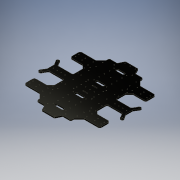
# Autodesk Inventor part: Acrylic Drivetrain Base - 1
Saved by Autodesk Inventor 2018 (Build 220112000, 112)
## iProperties
Created: 2018-08-24
Part Number: Acrylic Drivetrain Base - 1
Material: Generic
Document SubType Name: Modeling
Designer: anirudh
Density: 1 g/cm^3
Appearance: Gunmetal
Author: anirudh
Autodesk Inventor part; units mm, degrees
ref_plane "YZ Plane" through (0, 0, 0) normal (1, 0, 0) x (0, 1, 0)
ref_plane "XZ Plane" through (0, 0, 0) normal (0, 1, 0) x (-1, 0, 0)
ref_plane "XY Plane" through (0, 0, 0) normal (0, 0, 1) x (1, 0, 0)
sketch "Sketch1" plane through (0, 0, 0) normal (0, 1, 0) x (-1, 0, 0)
  line L0 (9.3096, -136.3312) -> (9.2955, -164.9037)
  circle A0 centre (71.6846, -205.4987) radius 1.85
  circle A1 centre (71.6846, -205.4987) radius 1.85
  circle A2 centre (156.9154, -205.4987) radius 1.85
  circle A3 centre (114.3, -205.4987) radius 1.85
  circle A4 centre (135.6077, -205.4987) radius 1.85
  circle A5 centre (92.9923, -205.4987) radius 1.85
  circle A6 centre (114.3, -256.2987) radius 1.85
  circle A7 centre (114.3, -307.0987) radius 1.85
  circle A8 centre (114.3, -357.8987) radius 1.85
  circle A9 centre (114.3, -403.3774) radius 1.85
  circle A10 centre (114.3, -205.4987) radius 1.85
  circle A11 centre (114.3, -154.6987) radius 1.85
  circle A12 centre (114.3, -103.8987) radius 1.85
  circle A13 centre (114.3, -53.0987) radius 1.85
  circle A14 centre (114.3, -7.62) radius 1.85
  circle A15 centre (31.75, -129.2987) radius 1.85
  circle A16 centre (31.75, -166.751) radius 1.85
  circle A17 centre (31.75, -92.7608) radius 1.85
  circle A18 centre (31.75, -281.6987) radius 1.85
  circle A19 centre (31.75, -244.2464) radius 1.85
  circle A20 centre (31.75, -318.2366) radius 1.85
  circle A21 centre (196.85, -129.2987) radius 1.85
  circle A22 centre (196.85, -166.751) radius 1.85
  circle A23 centre (196.85, -92.7608) radius 1.85
  circle A24 centre (196.85, -318.2366) radius 1.85
  circle A25 centre (196.85, -281.6987) radius 1.85
  circle A26 centre (196.85, -244.2464) radius 1.85
  line L1 (197.5093, -376.8271) -> (197.5095, -368.0768)
  line L2 (30.9869, -34.1675) -> (30.9883, -42.9178)
  line L3 (31.0103, -376.851) -> (31.011, -368.1007)
  line L4 (197.5254, -42.9116) -> (222.9296, -68.3074)
  line L5 (238.243, -117.2058) -> (219.1962, -136.2589)
  line L6 (219.1962, -274.5023) -> (238.2494, -293.5491)
  line L7 (222.9053, -342.6725) -> (197.5095, -368.0768)
  line L8 (5.6068, -342.705) -> (31.011, -368.1007)
  line L9 (-9.7544, -293.5747) -> (9.2924, -274.5216)
  line L10 (-9.7435, -117.2844) -> (9.3096, -136.3312)
  line L11 (5.5925, -68.322) -> (30.9883, -42.9178)
  arc A27 (158.3, -39.6917) -> (158.3, -43.3917) centre (158.3, -41.5417) ccw
  arc A28 (158.3, -167.6917) -> (158.3, -171.3917) centre (158.3, -169.5417) ccw
  circle A29 centre (139.7, -7.62) radius 1.85
  circle A30 centre (88.9, -7.62) radius 1.85
  circle A31 centre (139.7, -403.3774) radius 1.85
  circle A32 centre (88.9, -403.3774) radius 1.85
  circle A33 centre (156.9154, -182.6387) radius 1.85
  circle A34 centre (71.6846, -182.6387) radius 1.85
  circle A35 centre (156.9154, -228.3587) radius 1.85
  circle A36 centre (71.6846, -228.3587) radius 1.85
  circle A37 centre (144.8504, -332.4987) radius 1.85
  circle A38 centre (144.8504, -307.0987) radius 1.85
  circle A39 centre (144.8504, -281.6987) radius 1.85
  circle A40 centre (144.8504, -256.2987) radius 1.85
  circle A41 centre (144.8504, -354.6221) radius 1.85
  circle A42 centre (83.7496, -78.4987) radius 1.85
  circle A43 centre (83.7496, -103.8987) radius 1.85
  circle A44 centre (83.7496, -129.2987) radius 1.85
  circle A45 centre (83.7496, -154.6987) radius 1.85
  circle A46 centre (83.7496, -56.3753) radius 1.85
  circle A47 centre (83.7496, -281.6987) radius 1.85
  circle A48 centre (83.7496, -307.0987) radius 1.85
  circle A49 centre (83.7496, -332.4987) radius 1.85
  circle A50 centre (83.7496, -256.2987) radius 1.85
  circle A51 centre (196.85, -61.0108) radius 1.85
  circle A52 centre (196.85, -349.9866) radius 1.85
  circle A53 centre (31.75, -61.0108) radius 1.85
  circle A54 centre (31.75, -349.9866) radius 1.85
  arc A55 (124.9553, -184.4887) -> (124.9553, -180.7887) centre (124.9553, -182.6387) ccw
  arc A56 (124.9553, -230.2087) -> (124.9553, -226.5087) centre (124.9553, -228.3587) ccw
  arc A57 (103.6447, -180.7887) -> (103.6447, -184.4887) centre (103.6447, -182.6387) ccw
  arc A58 (103.6447, -226.5087) -> (103.6447, -230.2087) centre (103.6447, -228.3587) ccw
  line L12 (124.9553, -180.7887) -> (103.6447, -180.7887)
  line L13 (103.6447, -184.4887) -> (124.9553, -184.4887)
  line L14 (124.9553, -226.5087) -> (103.6447, -226.5087)
  line L15 (103.6447, -230.2087) -> (124.9553, -230.2087)
  circle A59 centre (222.9554, -81.0006) radius 1.85
  circle A60 centre (222.9554, -106.4006) radius 1.85
  circle A61 centre (205.7596, -112.7506) radius 1.85
  circle A62 centre (219.2568, -127.8041) radius 1.85
  circle A63 centre (222.9554, -329.9968) radius 1.85
  circle A64 centre (222.9554, -304.5968) radius 1.85
  circle A65 centre (205.7596, -298.2468) radius 1.85
  circle A66 centre (219.2568, -283.1933) radius 1.85
  circle A67 centre (5.6446, -81.0006) radius 1.85
  circle A68 centre (5.6446, -106.4006) radius 1.85
  circle A69 centre (22.8404, -112.7506) radius 1.85
  circle A70 centre (9.3432, -127.8041) radius 1.85
  circle A71 centre (22.8404, -298.2468) radius 1.85
  circle A72 centre (5.6446, -304.5968) radius 1.85
  circle A73 centre (5.6446, -329.9968) radius 1.85
  circle A74 centre (9.3432, -283.1933) radius 1.85
  circle A75 centre (15.5448, -164.846) radius 1.85
  circle A76 centre (15.5448, -246.1514) radius 1.85
  circle A77 centre (213.0552, -164.846) radius 1.85
  circle A78 centre (213.0552, -246.1514) radius 1.85
  line L16 (156.9471, -25.1432) -> (145.5867, -1.6614)
  arc A79 (197.5254, -34.1613) -> (191.1419, -27.8084) centre (191.1754, -34.1584) ccw
  arc A80 (145.5867, -1.6614) -> (142.9369, -0.0081) centre (142.9503, -2.9369) ccw
  arc A81 (156.9471, -25.1432) -> (160.8473, -27.8084) centre (161.2208, -23.0756) ccw
  line L17 (197.5093, -376.8271) -> (197.5095, -368.0768)
  line L18 (191.1555, -383.2007) -> (160.861, -383.2038)
  line L19 (156.961, -385.8694) -> (145.603, -409.3523)
  arc A82 (191.1555, -383.2007) -> (197.5093, -376.8271) centre (191.1593, -376.8507) ccw
  arc A83 (142.9534, -411.0059) -> (145.603, -409.3523) centre (142.9664, -408.0771) ccw
  arc A84 (160.861, -383.2038) -> (156.961, -385.8694) centre (161.2349, -387.9366) ccw
  line L20 (30.9869, -34.1675) -> (30.9883, -42.9178)
  line L21 (37.3358, -27.8164) -> (67.6304, -27.8114)
  line L22 (71.5302, -25.1455) -> (82.8866, -1.6618)
  arc A85 (37.3358, -27.8164) -> (30.9869, -34.1675) centre (37.3369, -34.1664) ccw
  arc A86 (85.5362, -0.0081) -> (82.8866, -1.6618) centre (85.5233, -2.9369) ccw
  arc A87 (67.6304, -27.8114) -> (71.5302, -25.1455) centre (67.2561, -23.0786) ccw
  arc A88 (31.0103, -376.851) -> (37.3598, -383.2016) centre (37.3603, -376.8516) ccw
  line L23 (37.3598, -383.2016) -> (67.6543, -383.2041)
  arc A89 (71.5543, -385.8697) -> (67.6543, -383.2041) centre (67.2805, -387.9369) ccw
  line L24 (71.5543, -385.8697) -> (82.9128, -409.3524)
  arc A90 (82.9128, -409.3524) -> (85.5625, -411.0059) centre (85.5493, -408.0771) ccw
  line L25 (9.2955, -164.9037) -> (9.2955, -171.2537)
  line L26 (5.5925, -68.322) -> (-60.4731, -68.322)
  line L27 (219.1962, -136.2589) -> (219.1962, -171.1839)
  line L28 (219.1962, -239.5772) -> (219.1962, -274.5023)
  line L29 (142.9534, -411.0059) -> (85.5625, -411.0059)
  line L30 (142.9369, -0.0081) -> (85.5362, -0.0081)
  line L31 (160.8473, -27.8084) -> (191.1419, -27.8084)
  line L32 (197.5254, -34.1613) -> (197.5254, -42.9116)
  line L33 (197.5254, -42.9116) -> (222.9296, -68.3074)
  line L34 (238.243, -117.2058) -> (219.2035, -136.2516)
  line L35 (-9.7435, -117.2844) -> (-61.6103, -117.2588)
  circle A91 centre (-85.9208, -164.4406) radius 1.85
  line L36 (-61.6103, -117.2588) -> (-37.1901, -117.2588) construction
  line L37 (-78.4107, -164.4544) -> (-65.7239, -184.4705)
  circle A92 centre (-85.9208, -246.5393) radius 1.85
  line L38 (-61.6326, -293.5491) -> (-37.2124, -293.5612) construction
  line L39 (-78.4057, -246.5412) -> (-65.7031, -226.5351)
  line L40 (-9.7544, -293.5747) -> (-61.6326, -293.5491)
  line L41 (-60.0894, -342.6725) -> (5.6068, -342.705)
  line L42 (-78.4057, -188.0789) -> (-78.4057, -222.901)
  line L43 (-91.143, -168.0218) -> (-78.4057, -188.0789)
  line L44 (-91.143, -242.9581) -> (-78.4057, -222.901)
  circle A93 centre (314.4543, -164.4406) radius 1.85
  line L45 (306.9417, -164.4412) -> (294.2391, -184.4473)
  line L46 (306.933, -246.5438) -> (294.2307, -226.5375)
  circle A94 centre (314.4543, -246.5393) radius 1.85
  line L47 (306.9392, -188.079) -> (306.9392, -222.901)
  line L48 (319.6764, -168.0218) -> (306.9392, -188.079)
  line L49 (319.6764, -242.9581) -> (306.9392, -222.901)
  line L50 (288.6229, -68.3074) -> (222.9296, -68.3074)
  line L51 (238.243, -117.2058) -> (290.1373, -117.2058)
  line L52 (290.1188, -293.5491) -> (238.2494, -293.5491)
  line L53 (222.9053, -342.6725) -> (288.6229, -342.6725)
  line L54 (-9.7435, -117.2844) -> (-61.6103, -117.2588)
  line L55 (-78.4107, -164.4544) -> (-65.7239, -184.4705)
  line L56 (-65.7031, -226.5351) -> (-78.4057, -246.5412)
  line L57 (-61.6326, -293.5491) -> (-9.7544, -293.5747)
  line L58 (238.243, -117.2058) -> (290.1373, -117.2058)
  line L59 (306.9417, -164.4412) -> (294.2391, -184.4473)
  line L60 (294.2307, -226.5375) -> (306.933, -246.5438)
  line L61 (290.1188, -293.5491) -> (238.2494, -293.5491)
  circle A95 centre (144.8375, -129.2857) radius 1.85
  circle A96 centre (144.8332, -103.8857) radius 1.85
  circle A97 centre (144.8289, -78.4857) radius 1.85
  circle A98 centre (144.8418, -154.6857) radius 1.85
  circle A99 centre (144.8251, -56.3623) radius 1.85
  arc A100 (159.225, -43.3917) -> (159.225, -39.6917) centre (159.225, -41.5417) ccw
  line L62 (159.225, -39.6917) -> (158.3, -39.6917)
  line L63 (158.3, -43.3917) -> (159.225, -43.3917)
  arc A101 (159.225, -171.3917) -> (159.225, -167.6917) centre (159.225, -169.5417) ccw
  line L64 (159.225, -167.6917) -> (158.3, -167.6917)
  line L65 (158.3, -171.3917) -> (159.225, -171.3917)
  arc A102 (158.3274, -367.5905) -> (158.328, -371.2905) centre (158.3277, -369.4405) ccw
  arc A103 (158.3058, -239.5905) -> (158.3064, -243.2905) centre (158.3061, -241.4405) ccw
  arc A104 (159.253, -371.2903) -> (159.2524, -367.5903) centre (159.2527, -369.4403) ccw
  line L66 (159.253, -371.2903) -> (158.328, -371.2905)
  line L67 (158.3274, -367.5905) -> (159.2524, -367.5903)
  arc A105 (159.2314, -243.2903) -> (159.2308, -239.5903) centre (159.2311, -241.4403) ccw
  line L68 (159.2314, -243.2903) -> (158.3064, -243.2905)
  line L69 (158.3058, -239.5905) -> (159.2308, -239.5903)
  arc A106 (70.2474, -43.3879) -> (70.2477, -39.6879) centre (70.2476, -41.5379) ccw
  arc A107 (70.2364, -171.3879) -> (70.2367, -167.6879) centre (70.2366, -169.5379) ccw
  arc A108 (69.3227, -39.6878) -> (69.3224, -43.3878) centre (69.3226, -41.5378) ccw
  line L70 (69.3227, -39.6878) -> (70.2477, -39.6879)
  line L71 (70.2474, -43.3879) -> (69.3224, -43.3878)
  arc A109 (69.3117, -167.6878) -> (69.3114, -171.3878) centre (69.3116, -169.5378) ccw
  line L72 (69.3117, -167.6878) -> (70.2367, -167.6879)
  line L73 (70.2364, -171.3879) -> (69.3114, -171.3878)
  line L74 (69.2988, -243.2864) -> (70.2238, -243.2867)
  arc A110 (69.2998, -239.5864) -> (69.2988, -243.2864) centre (69.2993, -241.4364) ccw
  line L75 (70.2248, -239.5867) -> (69.2998, -239.5864)
  arc A111 (69.2671, -367.5864) -> (69.2662, -371.2864) centre (69.2667, -369.4364) ccw
  line L76 (70.1921, -367.5867) -> (69.2671, -367.5864)
  line L77 (69.2662, -371.2864) -> (70.1912, -371.2867)
  arc A112 (70.2238, -243.2867) -> (70.2248, -239.5867) centre (70.2243, -241.4367) ccw
  arc A113 (70.1912, -371.2867) -> (70.1921, -367.5867) centre (70.1917, -369.4367) ccw
  line L78 (9.2955, -171.2537) -> (9.2955, -171.2643)
  line L79 (9.2924, -274.5216) -> (9.2924, -239.5943)
  circle A114 centre (-65.7031, -205.49) radius 1.85
  circle A115 centre (-46.6531, -205.49) radius 1.85
  circle A116 centre (-27.6031, -205.49) radius 1.85
  circle A117 centre (-8.5531, -205.49) radius 1.85
  circle A118 centre (294.2366, -205.5054) radius 1.85
  circle A119 centre (275.1866, -205.5038) radius 1.85
  circle A120 centre (256.1366, -205.5021) radius 1.85
  circle A121 centre (237.0866, -205.5005) radius 1.85
  line L80 (9.2924, -171.2627) -> (9.3096, -136.3312)
  line L81 (9.3096, -136.3312) -> (-9.7435, -117.2844)
  line L82 (-9.7435, -117.2844) -> (-61.6103, -117.2588)
  line L83 (-78.4107, -164.4544) -> (-65.7239, -184.4705)
  line L84 (9.2924, -171.2627) -> (9.3096, -136.3312)
  line L85 (-65.7696, -226.4913) -> (-78.4107, -246.5438)
  line L86 (-61.6326, -293.5491) -> (-9.7544, -293.5747)
  line L87 (-9.7544, -293.5747) -> (9.2924, -274.5216)
  line L88 (9.2924, -274.5216) -> (9.2924, -239.5943)
  line L89 (-60.4731, -68.322) -> (-61.6496, -68.322)
  line L90 (-71.1746, -77.847) -> (-71.1746, -107.7338)
  line L91 (-61.6496, -117.2588) -> (-61.6103, -117.2588)
  line L92 (-61.6496, -68.322) -> (-52.1246, -68.322)
  line L93 (-71.1746, -87.372) -> (-71.1746, -77.847)
  arc A122 (-61.6496, -68.322) -> (-71.1746, -77.847) centre (-61.6496, -77.847) ccw
  line L94 (-61.6496, -117.2588) -> (-52.1246, -117.2588)
  line L95 (-71.1746, -98.2088) -> (-71.1746, -107.7338)
  arc A123 (-71.1746, -107.7338) -> (-61.6496, -117.2588) centre (-61.6496, -107.7338) ccw
  line L96 (-87.0677, -156.6006) -> (-84.7607, -156.6006)
  line L97 (-78.4107, -162.9506) -> (-78.4107, -164.4544)
  line L98 (-87.0677, -254.3792) -> (-84.7607, -254.3792)
  line L99 (-78.4107, -248.0292) -> (-78.4107, -246.5438)
  line L100 (-71.1576, -303.0741) -> (-71.1576, -333.1475)
  line L101 (-60.0894, -342.6725) -> (-61.6326, -342.6725)
  line L102 (-61.6326, -293.5491) -> (-52.1076, -293.5491)
  line L103 (-71.1576, -312.5991) -> (-71.1576, -303.0741)
  line L104 (-61.6326, -342.6725) -> (-52.1076, -342.6725)
  line L105 (-71.1576, -323.6225) -> (-71.1576, -333.1475)
  arc A124 (-61.6279, -293.5491) -> (-71.1576, -303.0741) centre (-61.6326, -303.0741) ccw
  arc A125 (-71.1576, -333.1475) -> (-61.6326, -342.6725) centre (-61.6326, -333.1475) ccw
  line L106 (-65.7239, -184.4705) -> (2.9424, -184.4705)
  line L107 (9.2924, -178.1205) -> (9.2924, -171.2627)
  line L108 (-65.7696, -226.4913) -> (2.9424, -226.4913)
  line L109 (9.2924, -232.8413) -> (9.2924, -239.5943)
  line L110 (-93.0958, -164.9466) -> (-91.143, -168.0218)
  line L111 (-93.0958, -246.0333) -> (-91.143, -242.9581)
  line L112 (-87.0677, -156.6006) -> (-84.7607, -156.6006)
  line L113 (-87.0677, -156.6006) -> (-84.7607, -156.6006)
  arc A126 (-87.0677, -156.6006) -> (-93.0958, -164.9466) centre (-87.0677, -162.9506) ccw
  arc A127 (-78.4107, -162.9506) -> (-84.7607, -156.6006) centre (-84.7607, -162.9506) ccw
  line L114 (-78.4107, -246.5438) -> (-78.4107, -248.0292)
  arc A128 (-84.7607, -254.3792) -> (-78.4107, -248.0292) centre (-84.7607, -248.0292) ccw
  arc A129 (-93.0958, -246.0333) -> (-87.0677, -254.3792) centre (-87.0677, -248.0292) ccw
  line L115 (299.72, -326.2376) -> (299.72, -333.1475)
  line L116 (290.195, -342.6725) -> (288.6229, -342.6725)
  line L117 (299.72, -326.2376) -> (299.72, -303.0741)
  line L118 (290.195, -293.5491) -> (290.1188, -293.5491)
  line L119 (290.195, -342.6725) -> (280.67, -342.6725)
  line L120 (299.72, -323.6225) -> (299.72, -333.1475)
  arc A130 (290.195, -342.6725) -> (299.72, -333.1475) centre (290.195, -333.1475) ccw
  line L121 (290.195, -293.5491) -> (280.67, -293.5491)
  line L122 (299.72, -312.5991) -> (299.72, -303.0741)
  arc A131 (299.72, -303.0741) -> (290.195, -293.5491) centre (290.195, -303.0741) ccw
  line L123 (290.1373, -117.2058) -> (290.1994, -117.2058)
  line L124 (299.7244, -107.6808) -> (299.7244, -77.8324)
  line L125 (290.195, -68.3074) -> (288.6229, -68.3074)
  line L126 (290.1994, -117.2058) -> (280.6744, -117.2058)
  line L127 (299.7244, -98.1558) -> (299.7244, -107.6808)
  line L128 (290.195, -68.3074) -> (280.67, -68.3074)
  line L129 (299.7244, -87.3574) -> (299.7244, -77.8324)
  arc A132 (290.1994, -117.2058) -> (299.7244, -107.6808) centre (290.1994, -107.6808) ccw
  arc A133 (299.7244, -77.8324) -> (290.195, -68.3074) centre (290.1994, -77.8324) ccw
  line L130 (294.2307, -226.5375) -> (225.5462, -226.5375)
  line L131 (219.1962, -232.8875) -> (219.1962, -239.5772)
  line L132 (294.2391, -184.4473) -> (225.5462, -184.4473)
  line L133 (219.1962, -178.0973) -> (219.1962, -171.1839)
  line L134 (315.6011, -254.3793) -> (313.283, -254.3793)
  line L135 (306.933, -248.0293) -> (306.933, -246.5438)
  line L136 (321.6293, -246.0333) -> (319.6764, -242.9581)
  line L137 (306.9417, -164.4412) -> (306.9417, -162.968)
  line L138 (313.2917, -156.618) -> (315.6012, -156.618)
  line L139 (321.6411, -164.9279) -> (319.6764, -168.0218)
  arc A134 (315.6011, -254.3793) -> (321.6293, -246.0333) centre (315.6011, -248.0293) ccw
  line L140 (313.283, -254.3793) -> (315.6011, -254.3793)
  line L141 (306.933, -246.5438) -> (306.933, -248.0293)
  arc A135 (306.933, -248.0293) -> (313.283, -254.3793) centre (313.283, -248.0293) ccw
  line L142 (315.6012, -156.618) -> (313.2917, -156.618)
  arc A136 (321.6411, -164.9279) -> (315.6012, -156.618) centre (315.6012, -162.968) ccw
  line L143 (313.2917, -156.618) -> (315.6012, -156.618)
  line L144 (306.9417, -164.4412) -> (306.9417, -162.968)
  arc A137 (313.2917, -156.618) -> (306.9417, -162.968) centre (313.2917, -162.968) ccw
  line L145 (2.9424, -184.4705) -> (-3.4076, -184.4705)
  line L146 (9.2924, -171.7705) -> (9.2924, -178.1205)
  arc A138 (2.9424, -184.4705) -> (9.2924, -178.1205) centre (2.9424, -178.1205) ccw
  line L147 (2.9424, -226.4913) -> (-3.4076, -226.4913)
  line L148 (9.2924, -239.1913) -> (9.2924, -232.8413)
  arc A139 (9.2924, -232.8413) -> (2.9424, -226.4913) centre (2.9424, -232.8413) ccw
  line L149 (225.5462, -184.4473) -> (231.8962, -184.4473)
  line L150 (219.1962, -171.7473) -> (219.1962, -178.0973)
  line L151 (225.5462, -226.5375) -> (231.8962, -226.5375)
  line L152 (219.1962, -239.2375) -> (219.1962, -232.8875)
  arc A140 (219.1962, -178.0973) -> (225.5462, -184.4473) centre (225.5462, -178.0973) ccw
  arc A141 (225.5462, -226.5375) -> (219.1962, -232.8875) centre (225.5462, -232.8875) ccw
  circle A142 centre (196.85, -205.4987) radius 1.85
  circle A143 centre (31.75, -205.4987) radius 1.85
  circle A144 centre (290.195, -84.7598) radius 2.032
  circle A145 centre (290.195, -100.7618) radius 2.032
  circle A146 centre (258.191, -84.7598) radius 2.032
  circle A147 centre (258.191, -100.7618) radius 2.032
  circle A148 centre (290.195, -310.2356) radius 2.032
  circle A149 centre (290.195, -326.2376) radius 2.032
  circle A150 centre (258.191, -310.2356) radius 2.032
  circle A151 centre (258.191, -326.2376) radius 2.032
  circle A152 centre (-29.591, -310.2356) radius 2.032
  circle A153 centre (-29.591, -326.2376) radius 2.032
  circle A154 centre (-61.6085, -310.2203) radius 2.032
  circle A155 centre (-61.6106, -326.2223) radius 2.032
  circle A156 centre (-29.591, -84.7598) radius 2.032
  circle A157 centre (-29.591, -100.7618) radius 2.032
  circle A158 centre (-61.6106, -84.7576) radius 2.032
  circle A159 centre (-61.6085, -100.7596) radius 2.032
  circle A160 centre (83.7496, -354.6221) radius 1.85
  constraints: 306 end point, 161 centre point, 104 point on circle, 32 horizontal, 25 perpendicular, 17 collinear, 9 parallel, 8 vertical, 7 tangent, 2 point on line
ref_plane "Work Plane2" through (0, 6.35, 0) normal (0, 1, 0) x (1, 0, 0)
extrude "Extrusion21" add sketch "Sketch1" along normal blind 5.588
sketch "Sketch4" plane through (0, 5.588, 0) normal (0, 1, 0) x (1, 0, 0)
  circle A0 centre (-144.8251, 56.3623) radius 1.85 projected
  circle A1 centre (-83.7496, 56.3753) radius 1.85 projected
  circle A2 centre (-144.8418, 154.6857) radius 1.85 projected
  circle A3 centre (-83.7496, 154.6987) radius 1.85 projected
  circle A4 centre (-144.8504, 256.2987) radius 1.85 projected
  circle A5 centre (-83.7496, 256.2987) radius 1.85 projected
  circle A6 centre (-83.7496, 354.6221) radius 1.85 projected
  circle A7 centre (-144.8504, 354.6221) radius 1.85 projected
  arc A8 (-129.5313, 62.7155) -> (-129.5313, 50.0156) centre (-129.5532, 56.3656) ccw
  arc A9 (-99.0384, 50.0156) -> (-99.0384, 62.7155) centre (-99.0165, 56.3656) ccw
  arc A10 (-129.5313, 161.0421) -> (-129.5313, 148.3423) centre (-129.5709, 154.6922) ccw
  arc A11 (-99.0624, 148.3423) -> (-99.0624, 161.0421) centre (-99.0228, 154.6922) ccw
  arc A12 (-129.5313, 262.6485) -> (-129.5313, 249.9489) centre (-129.5752, 256.2987) ccw
  arc A13 (-99.0687, 249.9489) -> (-99.0687, 262.6485) centre (-99.0248, 256.2987) ccw
  arc A14 (-129.5313, 360.9719) -> (-129.5752, 348.2721) centre (-129.5752, 354.6221) ccw
  arc A15 (-99.0687, 348.2721) -> (-99.0687, 360.9719) centre (-99.0377, 354.622) ccw
  line L0 (-129.5752, 50.0156) -> (-99.0384, 50.0156)
  line L1 (-99.0384, 62.7155) -> (-129.5313, 62.7155)
  line L2 (-129.5313, 148.3423) -> (-99.0624, 148.3423)
  line L3 (-99.0624, 161.0421) -> (-129.5313, 161.0421)
  line L4 (-129.5313, 249.9489) -> (-99.0687, 249.9489)
  line L5 (-99.0687, 262.6485) -> (-129.5313, 262.6485)
  line L6 (-129.5752, 348.2721) -> (-99.0687, 348.2721)
  line L7 (-99.0687, 360.9719) -> (-129.5313, 360.9719)
  point P0 (0, 0)
  point P1 (-99.0248, 145.1672)
  dimension "d385" = 12.7
  dimension "d386" = 12.7
  dimension "d387" = 12.7
  dimension "d388" = 12.7
  dimension "d389" = 12.7
  dimension "d390" = 12.7
  dimension "d391" = 12.7
  dimension "d392" = 12.7
  constraints: 17 point on circle, 16 end point, 8 centre point, 7 parallel, 1 horizontal, 1 point on line, 1 tangent
  measures "d385" diameter of A8
  measures "d386" diameter of A9
  measures "d387" diameter of A10
  measures "d388" diameter of A11
  measures "d389" diameter of A12
  measures "d390" diameter of A13
  measures "d391" diameter of A14
  measures "d392" diameter of A15
extrude "Extrusion23" cut sketch "Sketch4" against normal blind 25.4 contours L1 A9 L0 A8 | L3 A11 L2 A10 | L5 A13 L4 A12 | L7 A15 L6 A14
sketch "Sketch5" plane through (0, 5.588, 0) normal (0, 1, 0) x (1, 0, 0)
  line L0 (-67.6304, 27.8114) -> (-37.3358, 27.8164) projected
  line L1 (-37.3358, 27.8164) -> (-30.9858, 27.8164)
  line L2 (-30.9869, 34.1675) -> (-30.9883, 42.9178) projected
  line L3 (-30.9858, 27.8164) -> (-30.9883, 42.9178)
  line L4 (-5.5925, 68.322) -> (61.6496, 68.322) projected
  line L5 (-30.9883, 42.9178) -> (-5.5925, 68.322)
  line L6 (9.7435, 117.2844) -> (-9.3096, 136.3312) projected
  line L7 (-9.2924, 232.8413) -> (-9.2924, 274.5216) projected
  line L8 (-9.2924, 274.5216) -> (-9.2924, 64.6209)
  line L9 (-9.2924, 274.5216) -> (9.7544, 293.5747) projected
  line L10 (-9.2924, 274.5216) -> (-9.2924, 346.3893)
  line L11 (-5.6068, 342.705) -> (-31.011, 368.1007) projected
  line L12 (-9.2924, 346.3893) -> (-31.011, 368.1007)
  line L13 (-31.011, 368.1007) -> (-31.0098, 383.201)
  line L14 (-37.3598, 383.2016) -> (-67.6543, 383.2041) projected
  line L15 (-31.0098, 383.201) -> (-37.3598, 383.2016)
  point P0 (0, 0)
  constraints: 16 end point, 3 collinear, 3 point on line, 2 perpendicular, 1 horizontal
body "Solid15"
